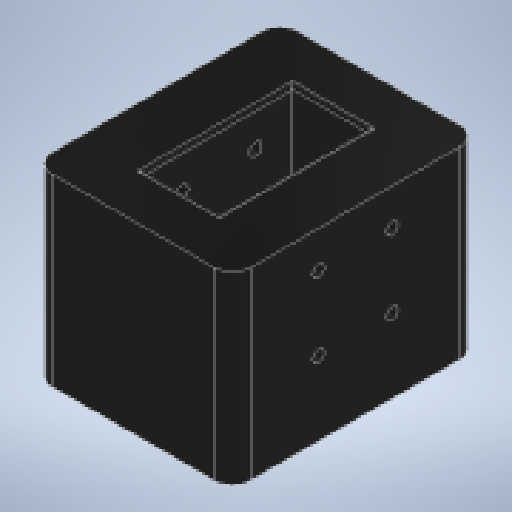
# Autodesk Inventor part: framefixpart1_v2
Saved by Autodesk Inventor 2024 (Build 280153000, 153)
## iProperties
Created: 2025-05-28
Part Number: framefixpart1_v2
Material: 一般
Document SubType Name: Modeling
Designer: kshau
Density: 1 g/cm^3
Appearance: 滑らか - 黒
Mass: 159.689 g
Surface Area: 260.007 cm^2
Volume: 159.689 cm^3
Author: kshau
Autodesk Inventor part; units mm, degrees
ref_plane "YZ Plane" through (0, 0, 0) normal (1, 0, 0) x (0, 1, 0)
ref_plane "XZ Plane" through (0, 0, 0) normal (0, 1, 0) x (-1, 0, 0)
ref_plane "XY Plane" through (0, 0, 0) normal (0, 0, 1) x (1, 0, 0)
sketch "スケッチ1" plane through (0, 0, 0) normal (0, 1, 0) x (-1, 0, 0)
  line L0 (0, 0) -> (54, 0)
  line L1 (54, 0) -> (54, -66.8)
  line L2 (54, -66.8) -> (0, -66.8)
  line L3 (0, -66.8) -> (0, 0)
  dimension "d0" = 54
  dimension "d1" = 66.8
  constraints: 8 end point, 2 parallel, 1 horizontal, 1 perpendicular
  measures "d0" distance of L0.start L0.end
  measures "d1" distance of L2.end L0.start
extrude "押し出し1" add sketch "スケッチ1" along normal blind 10
sketch "スケッチ2" plane through (0, 10, 0) normal (0, 1, 0) x (1, 0, 0)
  line L0 (-54, 66.8) -> (-54, 0) projected
  line L1 (-54, 0) -> (0, 0) projected
  line L2 (-27, 0) -> (-27, 66.8)
  line L3 (0, 66.8) -> (-54, 66.8) projected
  line L4 (-54, 33.4) -> (0, 33.4)
  line L5 (0, 0) -> (0, 66.8) projected
  line L6 (-27, 33.4) -> (-37.1, 33.4)
  line L7 (-37.1, 33.4) -> (-37.1, 53.5)
  line L8 (-37.1, 53.5) -> (-27, 53.5)
  line L9 (-27, 53.5) -> (-27, 33.4)
  line L10 (-37.1, 33.4) -> (-37.1, 13.3)
  line L11 (-37.1, 13.3) -> (-27, 13.3)
  line L12 (-16.9, 33.4) -> (-16.9, 53.5)
  line L13 (-16.9, 53.5) -> (-27, 53.5)
  line L14 (-16.9, 33.4) -> (-16.9, 13.3)
  line L15 (-16.9, 13.3) -> (-27, 13.3)
  dimension "d7" = 20.1
  dimension "d8" = 10.1
  constraints: 24 end point, 5 midpoint, 5 symmetric about line, 2 parallel, 1 horizontal, 1 perpendicular
  measures "d7" distance of L6.end L7.end
  measures "d8" distance of L7.end L8.end
extrude "押し出し2" add sketch "スケッチ2" along normal blind 40 contours L3 L2 L8 L7 L4 L0 | L4 L10 L11 L2 L1 L0 | L3 L5 L4 L12 L13 L2 | L2 L15 L14 L4 L5 L1
fillet "フィレット1" radius 5 4 edges at (0, 25, 0) (0, 25, -66.8) (-54, 25, -66.8) (-54, 25, 0)
sketch "スケッチ3" plane through (0, 0, -5) normal (1, 0, 0) x (0, 0, -1)
  line L0 (48.5, 50) -> (8.3, 50) projected
  line L1 (28.4, 50) -> (28.4, 0)
  line L2 (0, 0) -> (56.8, 0) projected
  line L3 (18.4, 50) -> (18.4, 0)
  line L4 (0, 50) -> (0, 0) projected
  line L5 (0, 10) -> (62, 10)
  line L6 (8.3, 10) -> (48.5, 10) projected
  point P0 (-5, 0)
  point P1 (18.4, 20)
  point P2 (18.4, 40)
  point P3 (38.4, 20)
  point P4 (38.4, 40)
  dimension "d12" = 10
  dimension "d13" = 10
  dimension "d14" = 10
  dimension "d15" = 20
  constraints: 6 end point, 3 point on line, 2 midpoint, 2 symmetric about line, 1 collinear, 1 vertical
  measures "d12" distance between parallel lines of L1 L3
  measures "d13" distance between parallel lines of L2 L5
  measures "d14" distance from line of L5 point (18.4, 20)
  measures "d15" distance of point (18.4, 20) point (18.4, 40)
hole "穴1" at (0, 20, -23.4) at (0, 40, -23.4) at (0, 40, -43.4) at (0, 20, -43.4) direction (-1, 0, 0) diameter 3.3 end through all
sketch "スケッチ4" plane through (0, 0, 0) normal (0, -1, 0) x (1, 0, 0)
  line L0 (-5, -66.8) -> (-49, -66.8) projected
  line L1 (-27, -66.8) -> (-27, 0)
  line L2 (-49, 0) -> (-5, 0) projected
  line L3 (-54, -61.8) -> (-54, -5) projected
  line L4 (-54, -33.4) -> (0, -33.4)
  line L5 (0, -5) -> (0, -61.8) projected
  point P0 (0, 0)
  point P1 (-27, -43.4)
  point P2 (-27, -23.4)
  dimension "d23" = 10
  dimension "d24" = 10
  constraints: 4 end point, 4 midpoint, 2 point on line
  measures "d23" distance from line of L4 point (-27, -23.4)
  measures "d24" distance from line of L4 point (-27, -43.4)
hole "穴2" at (-27, 0, -43.4) at (-27, 0, -23.4) direction (0, 1, 0) diameter 4.1 end through all
fillet "フィレット2" radius 1 4 edges at (-37.1, 50, -33.4) (-27, 50, -13.3) (-16.9, 50, -33.4) (-27, 50, -53.5)
sketch "スケッチ5" plane through (0, 0, 0) normal (0, -1, 0) x (1, 0, 0)
  circle A0 centre (-27, -23.4) radius 2.05 projected
  circle A1 centre (-27, -43.4) radius 2.05 projected
  line L0 (-27, -23.4) -> (-27, -43.4)
  line L1 (-27, -33.4) -> (-21, -33.4)
  line L2 (-21, -33.4) -> (-21, -39.4)
  line L3 (-21, -39.4) -> (-27, -39.4)
  line L4 (-27, -39.4) -> (-27, -33.4)
  line L5 (-21, -33.4) -> (-21, -27.4)
  line L6 (-21, -27.4) -> (-27, -27.4)
  line L7 (-33, -33.4) -> (-33, -39.4)
  line L8 (-33, -39.4) -> (-27, -39.4)
  line L9 (-33, -33.4) -> (-33, -27.4)
  line L10 (-33, -27.4) -> (-27, -27.4)
  point P0 (0, 0)
  dimension "d33" = 6
  dimension "d34" = 6
  constraints: 22 end point, 5 symmetric about line, 2 parallel, 1 horizontal, 1 midpoint, 1 perpendicular, 1 vertical
  measures "d33" distance of L1.end L2.end
  measures "d34" distance of L2.end L3.end
extrude "押し出し3" cut sketch "スケッチ5" against normal blind 10 contours L6 L5 L1 L0 | L0 L8 L7 L9 L10 | L1 L2 L3 L0
